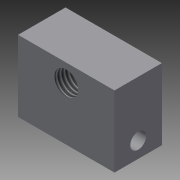
# Autodesk Inventor part: coupler
Saved by Autodesk Inventor 2015 (Build 190159000, 159)
## iProperties
Created: 2017-01-06
Part Number: coupler
Material: Generic
Document SubType Name: Modeling
Designer: ps2du
Density: 1 g/cm^3
Appearance: Default
Author: ps2du
Autodesk Inventor part; units mm, degrees
ref_plane "YZ Plane" through (0, 0, 0) normal (1, 0, 0) x (0, 1, 0)
ref_plane "XZ Plane" through (0, 0, 0) normal (0, 1, 0) x (-1, 0, 0)
ref_plane "XY Plane" through (0, 0, 0) normal (0, 0, 1) x (1, 0, 0)
sketch "Sketch1" plane through (0, 0, 0) normal (0, 0, 1) x (1, 0, 0)
  line L0 (0, 0) -> (38.735, 0)
  line L1 (38.735, 0) -> (38.735, 28.575)
  line L2 (38.735, 28.575) -> (0, 28.575)
  line L3 (0, 28.575) -> (0, 0)
  dimension "d0" = 38.735
  dimension "d1" = 28.575
  constraints: 8 end point, 2 parallel, 1 horizontal, 1 perpendicular
  measures "d0" distance of L2.end L1.end
  measures "d1" distance of L1.end L0.end
extrude "Extrusion1" add sketch "Sketch1" along normal blind 19.05
sketch "Sketch2" plane through (38.735, 0, 0) normal (1, 0, 0) x (0, 0, -1)
  line L0 (0, 0) -> (-19.05, 0)
  line L1 (0, 0) -> (-19.05, 0) projected
  line L2 (-19.05, 0) -> (-9.525, 0)
  line L3 (-9.525, 0) -> (-9.525, 28.575)
  line L4 (0, 28.575) -> (-19.05, 28.575) projected
  line L5 (-9.525, 0) -> (-9.525, 12.7)
  line L6 (-9.525, 12.7) -> (-9.525, 6.35)
  circle A0 centre (-9.525, 6.35) radius 3.175
  dimension "d4" = 12.7
  dimension "d5" = 6.35
  dimension "d6" = 6.35
  constraints: 10 end point, 3 midpoint, 1 centre point, 1 coincident, 1 collinear, 1 point on line
  measures "d4" distance of L2.end L5.end
  measures "d5" distance of L5.end L6.end
  measures "d6" diameter of A0
extrude "Extrusion2" cut sketch "Sketch2" against normal blind 76.2
sketch "Sketch3" plane through (0, 0, 19.05) normal (0, 0, 1) x (1, 0, 0)
  line L0 (0, 0) -> (0, 28.575)
  line L1 (0, 28.575) -> (0, 0) projected
  line L2 (0, 28.575) -> (38.735, 28.575)
  line L3 (38.735, 28.575) -> (19.3675, 28.575)
  line L4 (19.3675, 28.575) -> (19.3675, 0)
  line L5 (19.3675, 0) -> (19.3675, 14.2875)
  line L6 (19.3675, 14.2875) -> (19.3675, 28.575)
  line L7 (19.3675, 28.575) -> (19.3675, 21.4312)
  circle A0 centre (19.3675, 21.4312) radius 4.7625
  dimension "d9" = 9.525
  constraints: 14 end point, 3 midpoint, 2 collinear, 1 centre point, 1 coincident, 1 perpendicular, 1 vertical
  measures "d9" diameter of A0
extrude "Extrusion3" cut sketch "Sketch3" against normal blind 76.2
thread "Thread1" size "3/8-16 UNC" class "2B" standard "ANSI Unified Screw Threads" full length
body "Solid1"
